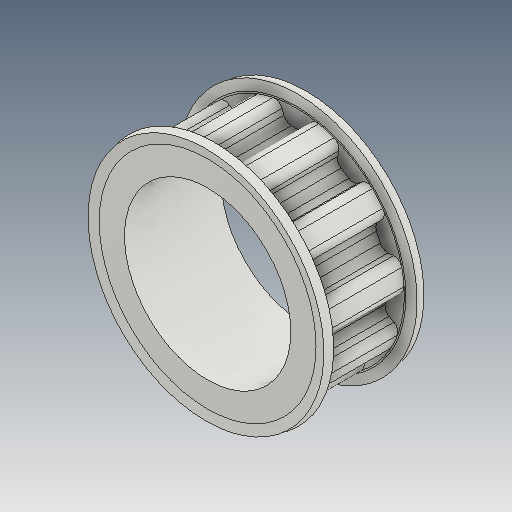
# Autodesk Inventor part: Synchronous Pulley2
Saved by Autodesk Inventor 2020.3 (Build 243373010, 373A)
## iProperties
CustomPartVersion: 1
Created: 2021-05-13
Part Number: Synchronous Pulley2
Material: Steel
Document SubType Name: Modeling
Designer: marti
Density: 1 g/cm^3
Appearance: Steel
Author: marti
Autodesk Inventor part; units mm, degrees
ref_plane "YZ Plane" through (0, 0, 0) normal (1, 0, 0) x (0, 1, 0)
ref_plane "XZ Plane" through (0, 0, 0) normal (0, 1, 0) x (-1, 0, 0)
ref_plane "XY Plane" through (0, 0, 0) normal (0, 0, 1) x (1, 0, 0)
sketch "Pulley Sketch" plane through (0, 0, 0) normal (0, 0, 1) x (1, 0, 0)
  circle A0 centre (0, 0) radius 16.6755 construction
  circle A1 centre (0, 0) radius 16.2945
  circle A2 centre (0, 0) radius 13.6275
  line L0 (-2.4285, 16.1125) -> (-1.524, 13.6275)
  line L1 (-1.524, 13.6275) -> (1.524, 13.6275)
  line L2 (1.524, 13.6275) -> (2.4285, 16.1125)
  line L3 (0, 0) -> (0, 16.2945) construction
  point P0 (0, 13.6275)
  dimension "d0" = 33.3509
  dimension "d1" = 0.381
  dimension "d2" = 2.667
  dimension "d3" = 40
  dimension "d4" = 3.048
  constraints: 8 end point, 3 coincident, 3 point on circle, 2 centre point, 1 horizontal, 1 midpoint, 1 point on line, 1 vertical, 1 vertical alignment, 3 other
  measures "d0" diameter of A0
  measures "d1" radial gap between concentric circles of A0 A1
  measures "d3" angle of L2 L0
  measures "d4" distance of L0.end L1.end
extrude "Base Body" add sketch "Pulley Sketch" along normal mid plane 12 contours A2 | A1 L0 L1 L2 | L2 L1 L0 A1
extrude "Tooth" cut sketch "Pulley Sketch" along normal through all both and the other way through all contours L2 L1 L0 A1 picked at (0, 15.392)
fillet "Tooth Fillet" radius 1.1938 2 edges at (1.524, 13.6275, 0) (-1.524, 13.6275, 0)
fillet "Tooth Fillet" radius 1.1684 4 edges at (-2.4285, 16.1125, 3) (-2.4285, 16.1125, -3) (2.4285, 16.1125, 3) (2.4285, 16.1125, -3)
pattern_circular "Teeth" count 11 over 360 about axis through (0, 0, -10) along (0, 0, 1) of "Tooth", "Tooth Fillet"
pulley flange "Left flange" diameter 32.5889 height 1.651 thickness 1.27 bend angle 10 centre (0, 0, -6) toward (0, 0, -1)
pulley flange "Right flange" diameter 32.5889 height 1.651 thickness 1.27 bend angle 10 centre (0, 0, 6) toward (0, 0, 1)
sketch "Sketch2" plane through (0, 0, 7.27) normal (0, 0, 1) x (1, 0, 0)
  circle A0 centre (0, 0) radius 12.5
  point P0 (0, 0)
  dimension "d17" = 25
  constraints: 1 centre point, 1 coincident
  measures "d17" diameter of A0
extrude "Extrusion3" cut sketch "Sketch2" against normal through all
equation "\"d1\" = da_a"
equation "\"d2\" = da_hg"
equation "\"d3\" = 2 * da_fi"
equation "\"d4\" = da_bw"
equation "\"d5\" = da_bf"
equation "\"d7\" = da_bf"
equation "\"d9\" = da_rb"
equation "\"d10\" = da_rt"
equation "\"da_pb\" = 9.525"
equation "\"da_fi\" = 20deg"
equation "\"da_hg\" = 2.667"
equation "\"da_bw\" = 3.048"
equation "\"da_rb\" = 1.1938"
equation "\"da_rt\" = 1.1684"
equation "\"da_a\" = 0.381"
equation "\"da_bf\" = 12"
equation "\"da_wf\" = 1.27"
equation "\"da_hf\" = 1.651"
body "Solid1"
